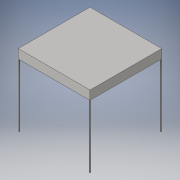
# Autodesk Inventor part: Pit
Saved by Autodesk Inventor 2016 SP2 (Build 200236200, 236)
## iProperties
Created: 2018-01-20
Part Number: Pit
Material: Generic
Document SubType Name: Modeling
Designer: CAD
Density: 1 g/cm^3
Appearance: Default
Author: CAD
Autodesk Inventor part; units mm, degrees
ref_plane "YZ Plane" through (0, 0, 0) normal (1, 0, 0) x (0, 1, 0)
ref_plane "XZ Plane" through (0, 0, 0) normal (0, 1, 0) x (-1, 0, 0)
ref_plane "XY Plane" through (0, 0, 0) normal (0, 0, 1) x (1, 0, 0)
sketch "Sketch1" plane through (0, 0, 0) normal (0, 0, 1) x (1, 0, 0)
  line L0 (0, 0) -> (0, 2438.4)
  line L1 (0, 2438.4) -> (2438.4, 2438.4)
  line L2 (2409.825, 2133.6) -> (28.575, 2133.6)
  line L3 (2438.4, 2438.4) -> (2438.4, 0)
  line L4 (2409.825, 0) -> (2409.825, 2133.6)
  line L5 (28.575, 2133.6) -> (28.575, 0)
  line L6 (0, 0) -> (28.575, 0)
  line L7 (2409.825, 0) -> (2438.4, 0)
  dimension "d0" = 0
  dimension "d1" = 2438.4
  dimension "d3" = 2438.4
  dimension "d4" = 304.8
  dimension "d5" = 28.575
  dimension "d7" = 28.575
  constraints: 16 end point, 2 horizontal, 1 collinear, 1 parallel, 1 vertical
  measures "d0" horizontal distance of L0.start L0.end
  measures "d1" distance of L0.start L0.end
  measures "d3" distance of L0.end L1.end
  measures "d4" distance between parallel lines of L1 L2
  measures "d5" distance between parallel lines of L3 L4
  measures "d7" distance between parallel lines of L0 L5
extrude "Extrusion1" add sketch "Sketch1" along normal blind 2438.4
sketch "Sketch2" plane through (2438.4, 0, 0) normal (1, 0, 0) x (0, 0, -1)
  line L0 (0, 2438.4) -> (-2438.4, 2438.4) projected
  line L1 (-2438.4, 0) -> (-2438.4, 2438.4) projected
  line L2 (0, 2438.4) -> (0, 0) projected
  line L3 (-2409.825, 0) -> (-2409.825, 2133.6)
  line L4 (-28.575, 2133.6) -> (-28.575, 0)
  line L5 (-2409.825, 2133.6) -> (-28.575, 2133.6)
  line L6 (0, 0) -> (-2438.4, 0) projected
  line L7 (-2409.825, 0) -> (-28.575, 0)
  dimension "d10" = 28.575
  dimension "d11" = 28.575
  dimension "d12" = 2133.6
  dimension "d13" = 2133.6
  dimension "d14" = 304.8
  constraints: 8 end point, 1 horizontal
  measures "d10" distance between parallel lines of L1 L3
  measures "d11" distance between parallel lines of L2 L4
  measures "d12" distance of L3.start L3.end
  measures "d13" distance of L4.start L4.end
  measures "d14" distance between parallel lines of L5 L0
extrude "Extrusion2" cut sketch "Sketch2" against normal blind 2438.4 contours L6 L3 L5 L4
sketch "Sketch3" plane through (28.575, 2133.6, 0) normal (0, -1, 0) x (1, 0, 0)
  line L0 (2381.25, 2409.825) -> (2381.25, 2438.4) projected
  line L1 (0, 2409.825) -> (0, 2438.4) projected
  line L2 (2381.25, 2409.825) -> (0, 2409.825)
  line L3 (0, 28.575) -> (-28.575, 28.575) projected
  line L4 (0, 2409.825) -> (0, 28.575)
  line L5 (0, 28.575) -> (2381.25, 28.575)
  line L6 (2381.25, 28.575) -> (2381.25, 2409.825)
  point P0 (-28.575, 0)
  constraints: 8 end point, 3 perpendicular, 1 horizontal
extrude "Extrusion3" cut sketch "Sketch3" against normal blind 276.225
body "Solid1"
